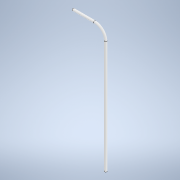
# Autodesk Inventor part: SP13V1 Tubo Baranda
Saved by Autodesk Inventor 2021.2 (Build 252289000, 289)
## iProperties
Created: 2026-05-19
Part Number: SP13V1 Tubo Baranda
Material: Acero, carbono
Document SubType Name: Modeling
Designer: nelso
Density: 7.85 g/cm^3
Appearance: Blanco
Author: nelso
Autodesk Inventor part; units mm, degrees
ref_plane "YZ Plane" through (0, 0, 0) normal (1, 0, 0) x (0, 1, 0)
ref_plane "XZ Plane" through (0, 0, 0) normal (0, 1, 0) x (-1, 0, 0)
ref_plane "XY Plane" through (0, 0, 0) normal (0, 0, 1) x (1, 0, 0)
sketch "Sketch1" plane through (0, 0, 0) normal (0, 1, 0) x (-1, 0, 0)
  circle A0 centre (0, 0) radius 15.55
  circle A1 centre (0, 0) radius 14.75
  dimension "d0" = 31.1
  dimension "d1" = 29.5
  constraints: 2 centre point, 2 coincident
  measures "d0" diameter of A0
  measures "d1" diameter of A1
sketch "Sketch2" plane through (0, 0, 0) normal (0, 0, 1) x (1, 0, 0)
  line L0 (-445, 1700) -> (-150, 1700)
  line L1 (0, 1550) -> (0, 0)
  arc A0 (0, 1550) -> (-150, 1700) centre (-150, 1550) ccw
  point P0 (0, 1700)
  dimension "d4" = 445
  dimension "d6" = 150
  dimension "d9" = 1700
  constraints: 4 end point, 2 point on circle, 2 point on line, 2 tangent, 1 centre point
  measures "d4" distance of L0.start point (0, 1700)
  measures "d6" radius of A0
  measures "d9" distance of point (0, 1700) L1.end
sweep "Sweep1" add profiles "Sketch1" path "Sketch2"
body "Solid2"
